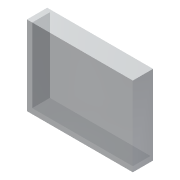
# Autodesk Inventor part: Vat
Saved by Autodesk Inventor 2014 (Build 180170000, 170)
## iProperties
Created: 2014-08-10
Part Number: Vat
Material: Generic
Document SubType Name: Modeling
Designer: Peele
Density: 1 g/cm^3
Appearance: Clear
Author: Peele
Autodesk Inventor part; units mm, degrees
ref_plane "YZ Plane" through (0, 0, 0) normal (1, 0, 0) x (0, 1, 0)
ref_plane "XZ Plane" through (0, 0, 0) normal (0, 1, 0) x (-1, 0, 0)
ref_plane "XY Plane" through (0, 0, 0) normal (0, 0, 1) x (1, 0, 0)
sketch "Sketch1" plane through (0, 0, 0) normal (0, 1, 0) x (-1, 0, 0)
  line L0 (-60, -45) -> (60, -45)
  line L1 (60, -45) -> (60, 45)
  line L2 (60, 45) -> (-60, 45)
  line L3 (-60, 45) -> (-60, -45)
  line L4 (-60, -45) -> (60, 45) construction
  line L5 (60, -45) -> (-60, 45) construction
  circle A0 centre (0, 0) radius 60 construction
  line L6 (40, -30) -> (0, -30) construction
  line L7 (0, -30) -> (0, 30) construction
  line L8 (0, 30) -> (40, 30) construction
  line L9 (40, 30) -> (40, -30) construction
  line L10 (40, -30) -> (0, 30) construction
  line L11 (0, -30) -> (40, 30) construction
  line L12 (-40, -30) -> (0, -30) construction
  line L13 (0, -30) -> (0, 30) construction
  line L14 (0, 30) -> (-40, 30) construction
  line L15 (-40, 30) -> (-40, -30) construction
  line L16 (-40, -30) -> (0, 30) construction
  line L17 (0, -30) -> (-40, 30) construction
  point P0 (20, 0)
  point P1 (-20, 0)
  point P2 (20, 0)
  point P3 (0, 0)
  point P4 (0, 0)
  dimension "d0" = 120
  dimension "d1" = 90
  dimension "d10" = 120
  dimension "d11" = 40
  dimension "d12" = 60
  constraints: 36 end point, 10 midpoint, 6 parallel, 3 horizontal, 3 perpendicular, 2 collinear, 1 centre point, 1 coincident, 1 horizontal alignment
  measures "d0" distance of L1.end L2.end
  measures "d1" distance of L0.end L1.end
  measures "d10" diameter of A0
  measures "d11" distance of L7.end L8.end
  measures "d12" distance of L8.end L6.start
extrude "Extrusion1" add sketch "Sketch1" along normal blind 3
sketch "Sketch2" plane through (0, 3, 0) normal (0, 1, 0) x (1, 0, 0)
  line L0 (60, 45) -> (-60, 45) projected
  line L1 (-60, 45) -> (-60, -45) projected
  line L2 (-60, -45) -> (60, -45)
  line L3 (60, -45) -> (60, 45)
  line L4 (60, 45) -> (-60, 45)
  line L5 (-60, 45) -> (-60, -45)
  line L6 (-60, -45) -> (60, 45) construction
  line L7 (60, -45) -> (-60, 45) construction
  line L8 (-57, -42) -> (57, -42)
  line L9 (57, -42) -> (57, 42)
  line L10 (57, 42) -> (-57, 42)
  line L11 (-57, 42) -> (-57, -42)
  line L12 (-57, -42) -> (57, 42) construction
  line L13 (57, -42) -> (-57, 42) construction
  point P0 (0, 0)
  point P1 (0, 0)
  dimension "d4" = 3
  dimension "d5" = 3
  constraints: 24 end point, 4 midpoint, 4 parallel, 2 horizontal, 2 perpendicular
  measures "d4" distance between parallel lines of L0 L10
  measures "d5" distance between parallel lines of L1 L11
extrude "Extrusion2" add sketch "Sketch2" along normal blind 20
body "Solid1"
